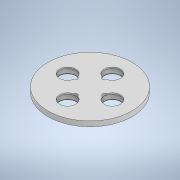
# Autodesk Inventor part: Крышка
Saved by Autodesk Inventor 2021.2 (Build 252289000, 289)
## iProperties
Created: 2021-07-30
Part Number: Крышка
Material: Типовые
Document SubType Name: Modeling
Designer: user
Density: 1 g/cm^3
Appearance: По умолчанию
Author: user
Autodesk Inventor part; units mm, degrees
ref_plane "YZ Plane" through (0, 0, 0) normal (1, 0, 0) x (0, 1, 0)
ref_plane "XZ Plane" through (0, 0, 0) normal (0, 1, 0) x (-1, 0, 0)
ref_plane "XY Plane" through (0, 0, 0) normal (0, 0, 1) x (1, 0, 0)
sketch "Эскиз1" plane through (0, 0, 0) normal (0, 1, 0) x (-1, 0, 0)
  circle A0 centre (0, 0) radius 75
  dimension "d0" = 150
  constraints: 1 centre point, 1 coincident
  measures "d0" diameter of A0
extrude "Выдавливание1" add sketch "Эскиз1" along normal blind 1
sketch "Эскиз2" plane through (0, 0, 0) normal (1, 0, 0) x (0, 1, 0)
  line L0 (0, 0) -> (0, 75)
  line L1 (0, 75) -> (-8, 75)
  line L2 (-8, 65) -> (0, 65)
  line L3 (-8, 75) -> (-8, 73.873)
  arc A0 (-8, 66.127) -> (-8, 73.873) centre (-9, 70) ccw
  line L4 (-8, 75) -> (-8, 73.873)
  line L5 (-8, 66.127) -> (-8, 65)
  line L6 (-11, 0) -> (3, 0) projected
  dimension "d3" = 75
  dimension "d4" = 8
  dimension "d5" = 10
  dimension "d8" = 8
  constraints: 12 end point, 2 point on circle, 2 vertical, 1 centre point, 1 horizontal, 1 point on line
  measures "d3" distance of L0.start L0.end
  measures "d4" distance of L0.end L1.end
  measures "d5" distance of L1.end L2.start
  measures "d8" diameter of A0
revolve "Вращение1" add sketch "Эскиз2" angle 360 about axis through (0, -10, 0) along (0, 1, 0)
sketch "Эскиз3" plane through (0, 1, 0) normal (0, 1, 0) x (1, 0, 0)
  circle A0 centre (0, 0) radius 39.907
  circle A1 centre (0, 39.907) radius 14.5
  circle A2 centre (39.907, 0) radius 14.5
  circle A3 centre (-39.907, 0) radius 14.5
  circle A4 centre (0, -39.907) radius 14.5
  dimension "d16" = 79.814
  dimension "d17" = 29
  dimension "d18" = 29
  dimension "d19" = 29
  dimension "d20" = 29
  constraints: 5 centre point, 4 point on circle, 1 coincident
  measures "d16" diameter of A0
  measures "d17" diameter of A1
  measures "d18" diameter of A2
  measures "d19" diameter of A3
  measures "d20" diameter of A4
extrude "Выдавливание2" cut sketch "Эскиз3" against normal blind 1 contours A0 A2 | A0 A2 | A1 A0 | A0 A1 | A4 A0 | A0 A4 | A3 A0 | A0 A3
sketch "Эскиз6" plane through (0, 1, 0) normal (0, 1, 0) x (1, 0, 0)
  circle A0 centre (0, 39.907) radius 14.5
  circle A1 centre (0, 39.907) radius 19.5
  circle A2 centre (39.907, 0) radius 14.5
  circle A3 centre (39.907, 0) radius 19.5
  circle A4 centre (0, -39.907) radius 19.5
  circle A5 centre (0, -39.907) radius 14.5
  circle A6 centre (-39.907, 0) radius 14.5
  circle A7 centre (-39.907, 0) radius 19.5
  point P0 (0, 0)
  dimension "d36" = 39
  dimension "d37" = 39
  dimension "d38" = 39
  dimension "d39" = 39
  constraints: 8 centre point, 4 coincident
  measures "d36" diameter of A1
  measures "d37" diameter of A3
  measures "d38" diameter of A4
  measures "d39" diameter of A7
extrude "Выдавливание3" add sketch "Эскиз6" against normal blind 11
sketch "Эскиз7" plane through (0, 0, 0) normal (1, 0, 0) x (0, 1, 0)
  line L0 (-1.127, -25.407) -> (-8.873, -25.407)
  line L1 (0, -20.407) -> (-10, -20.407) projected
  line L2 (-8.873, -25.407) -> (-5, -25.407)
  line L3 (1, -25.407) -> (-10, -25.407) projected
  arc A0 (-1.127, -25.407) -> (-8.873, -25.407) centre (-5, -26.407) ccw
  line L4 (3.2, -39.907) -> (-12.2, -39.907) projected
  point P0 (0, 0)
  constraints: 4 end point, 3 point on line, 2 point on circle, 1 centre point
revolve "Вращение2" cut sketch "Эскиз7" angle 360 about axis through (0, 1, -39.907) along (0, -1, 0)
sketch "Эскиз8" plane through (0, 0, 0) normal (1, 0, 0) x (0, 1, 0)
  line L0 (0, -75) -> (0, 75) projected
  line L1 (-1.127, 25.407) -> (-8.873, 25.407)
  line L2 (1, 25.407) -> (-10, 25.407) projected
  arc A0 (-8.873, 25.407) -> (-1.127, 25.407) centre (-5, 26.407) ccw
  line L3 (-12.2, 39.907) -> (3.2, 39.907) projected
  point P0 (0, 0)
  dimension "d52" = 8
  constraints: 2 end point, 2 point on circle, 1 centre point
  measures "d52" diameter of A0
revolve "Вращение3" cut sketch "Эскиз8" angle 360 about axis through (0, 0, 39.907) along (0, 1, 0)
sketch "Эскиз9" plane through (0, 0, 0) normal (0, 0, 1) x (1, 0, 0)
  line L0 (75, 0) -> (-75, 0) projected
  line L1 (25.407, -1.127) -> (25.407, -8.873)
  line L2 (25.407, -5) -> (26.407, -5)
  arc A0 (25.407, -1.127) -> (25.407, -8.873) centre (26.407, -5) ccw
  line L3 (39.907, -10.8476) -> (39.907, 2.9746) projected
  point P0 (0, 0)
  dimension "d57" = 1
  dimension "d58" = 8
  constraints: 4 end point, 2 point on circle, 1 centre point, 1 coincident, 1 midpoint, 1 perpendicular
  measures "d57" distance of L2.start L2.end
  measures "d58" diameter of A0
revolve "Вращение4" cut sketch "Эскиз9" angle 360 about axis through (39.907, 0, 0) along (0, 1, 0)
sketch "Эскиз10" plane through (0, 0, 0) normal (0, 0, 1) x (1, 0, 0)
  line L0 (75, 0) -> (-75, 0) projected
  line L1 (-25.407, -1.127) -> (-25.407, -8.873)
  line L2 (-25.407, -5) -> (-26.407, -5)
  arc A0 (-25.407, -8.873) -> (-25.407, -1.127) centre (-26.407, -5) ccw
  line L3 (-39.907, 3.2) -> (-39.907, -12.2) projected
  point P0 (0, 0)
  dimension "d63" = 1
  dimension "d64" = 8
  constraints: 4 end point, 2 point on circle, 1 centre point, 1 coincident, 1 midpoint, 1 vertical
  measures "d63" distance of L2.start L2.end
  measures "d64" diameter of A0
revolve "Вращение5" cut sketch "Эскиз10" angle 360 about axis through (-39.907, 1, 0) along (0, -1, 0)
sketch "Эскиз11" plane through (0, -10, 39.907) normal (0, -1, 0) x (1, 0, 0)
  circle A0 centre (0, 0) radius 115.9174
  point P0 (0, -39.907)
  constraints: 1 centre point
extrude "Выдавливание4" cut sketch "Эскиз11" against normal blind 0.5
sketch "Эскиз12" plane through (0, 1, 0) normal (0, 1, 0) x (1, 0, 0)
  line L0 (0, 0) -> (0, -26.407)
  line L1 (0, 0) -> (-26.407, 0)
  line L2 (0, 0) -> (0, 26.407)
  line L3 (0, 0) -> (26.407, 0)
  circle A0 centre (0, -26.407) radius 4
  circle A1 centre (-26.407, 0) radius 4
  circle A2 centre (0, 26.407) radius 4
  circle A3 centre (26.407, 0) radius 4
  dimension "d68" = 26.407
  dimension "d69" = 26.407
  dimension "d70" = 26.407
  dimension "d71" = 26.407
  dimension "d72" = 8
  dimension "d73" = 8
  dimension "d74" = 8
  dimension "d75" = 8
  constraints: 8 end point, 4 centre point, 4 coincident, 2 horizontal, 2 vertical
  measures "d68" distance of L0.start L0.end
  measures "d69" distance of L0.start L1.end
  measures "d70" distance of L0.start L2.end
  measures "d71" distance of L0.start L3.end
  measures "d72" diameter of A0
  measures "d73" diameter of A1
  measures "d74" diameter of A2
  measures "d75" diameter of A3
extrude "Выдавливание5" cut sketch "Эскиз12" against normal blind 5
